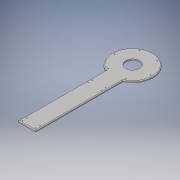
# Autodesk Inventor part: Arm Layer 1
Saved by Autodesk Inventor 2016 (Build 200138000, 138)
## iProperties
Created: 2016-04-16
Part Number: Arm Layer 1
Material: Generic
Document SubType Name: Modeling
Designer: rmarkowi
Density: 1 g/cm^3
Appearance: Default
Author: rmarkowi
Autodesk Inventor part; units mm, degrees
ref_plane "YZ Plane" through (0, 0, 0) normal (1, 0, 0) x (0, 1, 0)
ref_plane "XZ Plane" through (0, 0, 0) normal (0, 1, 0) x (-1, 0, 0)
ref_plane "XY Plane" through (0, 0, 0) normal (0, 0, 1) x (1, 0, 0)
sketch "Sketch1" plane through (0, 0, 0) normal (0, 1, 0) x (-1, 0, 0)
  line L0 (0, 0) -> (152.4, 0)
  line L1 (152.4, 0) -> (152.4, -762)
  line L2 (0, -762) -> (0, 0)
  line L3 (152.4, -762) -> (0, -762) construction
  arc A0 (0, -762) -> (152.4, -762) centre (76.2, -922.6437) ccw
  line L4 (152.4, -590.1365) -> (152.4, -762) construction
  circle A1 centre (76.2, -922.6437) radius 60.325
  dimension "d1" = 762
  dimension "d5" = 355.6
  dimension "d6" = 120.65
  dimension "d11" = 762
  constraints: 10 end point, 2 centre point, 2 point on circle, 1 coincident, 1 collinear, 1 horizontal, 1 parallel, 1 perpendicular, 1 point on line
  measures "d1" distance of L0.end L1.end
  measures "d5" diameter of A0
  measures "d6" diameter of A1
  measures "d11" distance of L2.start L0.start
extrude "Extrusion1" add sketch "Sketch1" along normal blind 12.7
fillet "Fillet1" radius 6.35 4 edges at (-76.2, 12.7, 0) (0, 12.7, -381) (-152.4, 12.7, -381) (-76.2, 12.7, -1100.4437)
sketch "Sketch2" plane through (0, 12.7, 0) normal (0, 1, 0) x (1, 0, 0)
  circle A0 centre (-76.2, 922.6437) radius 60.325 construction
  line L0 (-76.2, 922.6437) -> (-76.2, 862.3187) construction
  circle A1 centre (-76.2, 922.6437) radius 157.48 construction
  circle A2 centre (-233.68, 922.6437) radius 3.81
  circle A3 centre (-154.94, 786.262) radius 3.81
  circle A4 centre (2.54, 786.262) radius 3.81
  circle A5 centre (81.28, 922.6437) radius 3.81
  circle A6 centre (2.54, 1059.0254) radius 3.81
  circle A7 centre (-154.94, 1059.0254) radius 3.81
  point P0 (0, 0)
  dimension "d10" = 314.96
  dimension "d12" = 7.62
  dimension "d15" = 360
  constraints: 6 centre point, 2 end point, 1 coincident, 1 horizontal alignment, 1 vertical, 1 vertical alignment, 16 other
  measures "d12" diameter of A2
extrude "Extrusion2" cut sketch "Sketch2" against normal blind 12.7
sketch "Sketch3" plane through (0, 12.7, 0) normal (0, 1, 0) x (1, 0, 0)
  line L0 (0, 0) -> (-152.4, 0) construction
  line L1 (-76.2, 0) -> (-76.2, 12.7) construction
  line L2 (-76.2, 0) -> (-63.5, 0) construction
  line L3 (-12.7, 15.875) -> (-12.7, 60.325) construction
  line L4 (-15.875, 63.5) -> (-136.525, 63.5) construction
  line L5 (-139.7, 60.325) -> (-139.7, 15.875) construction
  line L6 (-136.525, 12.7) -> (-15.875, 12.7) construction
  circle A0 centre (-19.05, 57.15) radius 3.175
  circle A1 centre (-19.05, 57.15) radius 3.175
  circle A2 centre (-19.05, 19.05) radius 3.175
  circle A3 centre (-19.05, 19.05) radius 3.175
  circle A4 centre (-133.35, 57.15) radius 3.175
  circle A5 centre (-133.35, 57.15) radius 3.175
  circle A6 centre (-133.35, 19.05) radius 3.175
  arc A7 (-12.7, 60.325) -> (-15.875, 63.5) centre (-15.875, 60.325) ccw construction
  arc A8 (-15.875, 12.7) -> (-12.7, 15.875) centre (-15.875, 15.875) ccw construction
  arc A9 (-139.7, 15.875) -> (-136.525, 12.7) centre (-136.525, 15.875) ccw construction
  arc A10 (-136.525, 63.5) -> (-139.7, 60.325) centre (-136.525, 60.325) ccw construction
  line L7 (-76.2, 12.7) -> (-76.2, 63.5) construction
  line L8 (-76.2, 63.5) -> (-76.2, 584.2) construction
  line L9 (-139.7, 676.656) -> (-104.4, 676.656) construction
  line L10 (-139.7, 676.656) -> (-139.7, 587.375) construction
  line L11 (-136.525, 584.2) -> (-15.875, 584.2) construction
  line L12 (-12.7, 587.375) -> (-12.7, 676.656) construction
  line L13 (-12.7, 676.656) -> (-139.7, 676.656) construction
  arc A11 (-139.7, 587.375) -> (-136.525, 584.2) centre (-136.525, 587.375) ccw construction
  arc A12 (-15.875, 584.2) -> (-12.7, 587.375) centre (-15.875, 587.375) ccw construction
  circle A13 centre (-133.35, 590.55) radius 3.175
  circle A14 centre (-133.35, 590.55) radius 3.175
  circle A15 centre (-133.35, 628.65) radius 3.175
  circle A16 centre (-133.35, 628.65) radius 3.175
  circle A17 centre (-19.05, 590.55) radius 3.175
  circle A18 centre (-19.05, 590.55) radius 3.175
  circle A19 centre (-19.05, 628.65) radius 3.175
  circle A20 centre (-19.05, 628.65) radius 3.175
  line L14 (-76.2, 584.2) -> (-76.2, 676.656) construction
  point P0 (-12.7, 12.7)
  point P1 (-139.7, 635)
  dimension "d19" = 12.7
  dimension "d20" = 90
  dimension "d21" = 3.175
  dimension "d24" = 520.7
  dimension "d26" = 3.175
  constraints: 28 end point, 21 centre point, 15 coincident, 12 point on circle, 12 tangent, 5 midpoint, 4 equal radius, 4 parallel, 3 perpendicular, 2 point on line, 2 vertical, 1 horizontal
  measures "d19" distance of L1.start L1.end
  measures "d20" angle of L2 L1
  measures "d21" radius of A7
  measures "d24" distance of L7.end L8.end
  measures "d26" radius of A11
extrude "Extrusion3" cut sketch "Sketch3" against normal blind 12.7
body "Solid1"
